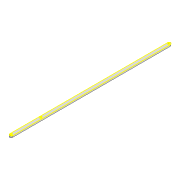
# Autodesk Inventor part: Wing_arm_2
Saved by Autodesk Inventor 2022 (Build 260153000, 153)
## iProperties
Created: 2022-07-07
Part Number: Wing_arm_2
Material: Generic
Document SubType Name: Modeling
Designer: dell
Density: 1 g/cm^3
Appearance: Default
Author: dell
Autodesk Inventor part; units mm, degrees
ref_plane "YZ Plane" through (0, 0, 0) normal (1, 0, 0) x (0, 1, 0)
ref_plane "XZ Plane" through (0, 0, 0) normal (0, 1, 0) x (-1, 0, 0)
ref_plane "XY Plane" through (0, 0, 0) normal (0, 0, 1) x (1, 0, 0)
sketch "Sketch1" plane through (0, 0, 0) normal (0, 1, 0) x (-1, 0, 0)
  line L0 (0, 0) -> (0, -411.151) construction
  line L1 (-4, 0) -> (-4, -411.151)
  line L2 (4, -411.151) -> (4, 0)
  arc A0 (4, 0) -> (-4, 0) centre (0, 0) ccw
  arc A1 (-4, -411.151) -> (4, -411.151) centre (0, -411.151) ccw
  circle A2 centre (0, -411.151) radius 1.5
  circle A3 centre (0, 0) radius 1.5
  circle A4 centre (0, -77.048) radius 1.5
  point P0 (0, -205.5755)
  dimension "d0" = 411.151
  dimension "d1" = 8
  dimension "d2" = 3
  dimension "d3" = 3
  dimension "d6" = 3
  dimension "d7" = 334.103
  constraints: 8 end point, 5 centre point, 4 point on circle, 4 tangent, 2 coincident, 1 midpoint, 1 parallel, 1 point on line, 1 vertical
  measures "d0" distance of L0.start L0.end
  measures "d1" diameter of A1
  measures "d2" diameter of A2
  measures "d3" diameter of A3
  measures "d6" diameter of A4
  measures "d7" distance of L0.end A4.centre
extrude "Extrusion1" add sketch "Sketch1" along normal blind 4.5
sketch "Sketch2" plane through (0, 4.5, 0) normal (0, 1, 0) x (1, 0, 0)
  arc A0 (4, 411.151) -> (-4, 411.151) centre (0, 411.151) ccw projected
  line L0 (-4, 411.151) -> (-4, 0) projected
  arc A1 (-4, 0) -> (4, 0) centre (0, 0) ccw projected
  line L1 (4, 0) -> (4, 411.151) projected
  circle A2 centre (0, 77.048) radius 1.5 projected
  circle A3 centre (0, 0) radius 1.5 projected
  circle A4 centre (0, 411.151) radius 1.5 projected
body "Solid1"
